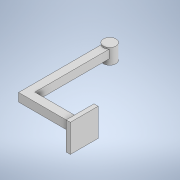
# Autodesk Inventor part: socket
Saved by Autodesk Inventor 2020.2 (Build 242310000, 310)
## iProperties
Created: 2020-02-07
Part Number: socket
Material: Generic
Document SubType Name: Modeling
Designer: ColinP
Density: 1 g/cm^3
Appearance: Default
Author: ColinP
Autodesk Inventor part; units mm, degrees
ref_plane "YZ Plane" through (0, 0, 0) normal (1, 0, 0) x (0, 1, 0)
ref_plane "XZ Plane" through (0, 0, 0) normal (0, 1, 0) x (-1, 0, 0)
ref_plane "XY Plane" through (0, 0, 0) normal (0, 0, 1) x (1, 0, 0)
sketch "Sketch3" plane through (0, 0, 0) normal (0, 1, 0) x (-1, 0, 0)
  circle A0 centre (0, 0) radius 4.5
  circle A1 centre (0, 0) radius 2.6
  dimension "d10" = 9
  dimension "d11" = 5.2
  constraints: 2 centre point, 2 coincident
  measures "d10" diameter of A0
  measures "d11" diameter of A1
extrude "Extrusion2" add sketch "Sketch3" along normal blind 4
sketch "Sketch4" plane through (0, 4, 0) normal (0, 1, 0) x (1, 0, 0)
  circle A0 centre (0, 0) radius 2.6 projected
  line L0 (0, -2.6) -> (0, -1.6)
  line L1 (0, -1.6) -> (0, 2.6)
  line L2 (0, -1.6) -> (-2.0494, -1.6)
  line L3 (0, -1.6) -> (2.0494, -1.6)
  line L4 (0, 2.6) -> (0, 2.6)
  line L5 (0, 2.6) -> (0, 2.6)
  circle A1 centre (0, 0) radius 4.5 projected
  circle A2 centre (0, 0) radius 2.6 projected
  line L6 (0, 2.6) -> (0, 1.6)
  line L7 (0, 1.6) -> (2.0494, 1.6)
  line L8 (0, 1.6) -> (-2.0494, 1.6)
  point P0 (2.0494, 1.6)
  point P1 (-2.0494, 1.6)
  dimension "d14" = 1
  dimension "d20" = 1
  constraints: 18 end point, 7 point on circle, 4 point on line, 1 horizontal, 1 midpoint, 1 parallel, 1 perpendicular, 1 vertical
  measures "d14" distance of L0.start L0.end
  measures "d20" distance of L5.end L6.end
extrude "Extrusion3" add sketch "Sketch4" along normal blind 6 contours L7 L1 A0 | A0 L0 L3 | L1 L8 A0 | A0 L2 L0 | A1
sketch "Sketch5" plane through (0, 10, 0) normal (0, 1, 0) x (1, 0, 0)
  circle A0 centre (0, 0) radius 4.5 projected
extrude "Extrusion4" add sketch "Sketch5" along normal blind 1
sketch "Sketch6" plane through (2.0494, 4, 1.6) normal (0, 0, -1) x (-1, 0, 0)
  line L0 (4.0988, 6) -> (0, 6) projected
  line L1 (2.0494, 6) -> (2.0494, 3)
  line L2 (2.0494, 6) -> (5.0494, 6) construction
  line L3 (2.0494, 6) -> (-0.9506, 6)
  line L4 (2.0494, 6) -> (5.0494, 6) construction
  line L5 (-0.9506, 6) -> (-0.9506, 0)
  line L6 (-0.9506, 0) -> (5.0494, 0)
  line L7 (5.0494, 0) -> (5.0494, 6)
  line L8 (5.0494, 6) -> (-0.9506, 6)
  line L9 (4.6494, 6) -> (4.6494, -4) projected
  point P0 (2.0494, -4)
  point P1 (4.6494, 0)
  point P2 (0, 6)
  dimension "d21" = 3
  dimension "d22" = 90
  dimension "d32" = 3
  dimension "d33" = 180
  dimension "d34" = 6
  dimension "d35" = 90
  dimension "d36" = 6
  dimension "d37" = 90
  constraints: 16 end point, 3 horizontal, 3 perpendicular, 2 equal length, 1 midpoint, 1 vertical
  measures "d21" distance of L1.start L1.end
  measures "d22" angle of L1 L2
  measures "d32" distance of L1.start L3.end
  measures "d33" angle of L3 L4
  measures "d34" distance of L3.end L5.end
  measures "d35" angle of L5 L3
  measures "d36" distance of L5.end L6.end
  measures "d37" angle of L6 L5
extrude "Extrusion7" add sketch "Sketch6" against normal blind 61.2 contours L8 L9 L6 L5 L3 L0
sketch "Sketch8" plane through (3, 4, 3.3541) normal (1, 0, 0) x (0, 0, -1)
  line L0 (-0.3188, 6) -> (-59.4459, 6) projected
  line L1 (-59.4459, 6) -> (-53.4459, 6)
  line L2 (-53.4459, 6) -> (-53.4459, 0)
  line L3 (-0.3188, 0) -> (-59.4459, 0) projected
  line L4 (0, 6) -> (0, 0) projected
  line L5 (0, 6) -> (-59.4459, 6) projected
  line L6 (-59.4459, 0) -> (-59.4459, 6) projected
  line L7 (0, 0) -> (-59.4459, 0) projected
  point P0 (3.3541, -4)
  dimension "d40" = 6
  constraints: 4 end point, 2 point on line, 1 perpendicular
  measures "d40" distance of L0.end L1.end
extrude "Extrusion8" add sketch "Sketch8" along normal blind 35.56 contours L2 L3 L6 L0
sketch "Sketch11" plane through (38.56, 4, 3.3541) normal (1, 0, 0) x (0, 0, -1)
  line L0 (-59.4459, 6) -> (-59.4459, 0) projected
  line L1 (-59.4459, 6) -> (-66.4436, 6)
  line L2 (-66.4436, 6) -> (-66.4436, 13.0104)
  line L3 (-66.4436, 13.0104) -> (-59.4459, 13.0104)
  line L4 (-59.4459, 13.0104) -> (-59.4459, 6)
  line L5 (-66.4436, 13.0104) -> (-46.4538, 13.0104)
  line L6 (-46.4538, 13.0104) -> (-46.4538, -6.9794)
  line L7 (-46.4538, -6.9794) -> (-66.4436, -6.9794)
  line L8 (-66.4436, -6.9794) -> (-66.4436, 13.0104)
  point P0 (3.3541, -4)
  dimension "d59" = 6.9977
  dimension "d60" = 7.0104
  dimension "d61" = 19.9898
  dimension "d62" = 19.9898
  constraints: 16 end point, 4 parallel, 2 horizontal, 2 perpendicular
  measures "d59" distance of L2.end L3.end
  measures "d60" distance of L1.end L2.end
  measures "d61" distance of L6.end L7.end
  measures "d62" distance of L5.end L6.end
extrude "Extrusion11" add sketch "Sketch11" along normal blind 3
body "Solid2"
